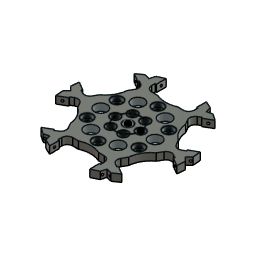
Omni_1 (Autodesk Fusion 360 design; units mm, degrees)
Autodesk Fusion 360 part; units mm, degrees
sketch "Sketch2" plane through (0, 0, 0) normal (0, 1, 0) x (1, 0, 0)
  line L0 (11.1, 32.1629) -> (11.1, 26.801)
  line L1 (-11.1, 26.801) -> (-11.1, 32.1629)
  line L2 (-11.1, 26.801) -> (-11.75, 26.801)
  line L3 (11.1, 26.801) -> (11.75, 26.801)
  line L4 (0, 0) -> (-15.82, 27.401)
  line L5 (0, 0) -> (15.82, 27.401)
  line L6 (0, 0) -> (0, 55) construction
  line L7 (15.82, 27.401) -> (15.0435, 30.2988)
  line L8 (-15.82, 27.401) -> (-15.0435, 30.2988)
  line L9 (-15.0435, 30.2988) -> (-11.1, 32.1629)
  line L10 (15.0435, 30.2988) -> (11.1, 32.1629)
  line L11 (-11.75, 26.801) -> (-11.75, 24.801)
  line L12 (11.75, 26.801) -> (11.75, 24.801)
  line L13 (-8.7379, 21.8005) -> (-5.5379, 21.8005)
  line L14 (8.7379, 21.8005) -> (5.5379, 21.8005)
  arc A0 (-11.75, 24.801) -> (-8.7379, 21.8005) centre (-8.75, 24.8004) ccw
  arc A1 (-5.5379, 21.8005) -> (5.5379, 21.8005) centre (0, 33.7826) ccw
  arc A2 (8.7379, 21.8005) -> (11.75, 24.801) centre (8.75, 24.8004) ccw
  circle A3 centre (0, 16.5) radius 1.64
  point P0 (0.1, 26.7998)
  dimension "d41" = 26.8
  dimension "d43" = 11
  dimension "d45" = 0.65
  dimension "d46" = 60
  dimension "d47" = 30
  dimension "d48" = 31.64
  dimension "d49" = 0.6
  dimension "d50" = 0.6
  dimension "d51" = 135
  dimension "d52" = 135
  dimension "d53" = 3
  dimension "d54" = 3
  dimension "d55" = 2
  dimension "d56" = 2
  dimension "d63" = 6
  dimension "d64" = 3
  dimension "d65" = 6
  dimension "d66" = 3
  dimension "d67" = 3.2
  dimension "d68" = 3.2
  dimension "d69" = 26.4
  dimension "d70" = 3.28
  dimension "d71" = 16.5
  dimension "d82" = 11.1
  dimension "d83" = 11.1
  constraint vertical L0
  constraint vertical L1
  constraint perpendicular L1 L2
  constraint perpendicular L0 L3
  constraint equal L2 L3
  constraint coincident L4.start L5.start
  constraint vertical L6
  constraint equal L4 L5
  constraint perpendicular L2 L11
  constraint perpendicular L3 L12
  constraint perpendicular L1 L13
  constraint horizontal L14
  constraint coincident L6 A3.centre
  measures "d41" distance of L4.start P0
  measures "d43" distance of L0 P0
  measures "d45" distance of L1.start L2.end
  measures "d46" angle of L4 L5
  measures "d47" angle of L5 L6
  measures "d48" distance of L4.start L4.end
  measures "d49" distance of L2 L4.end
  measures "d50" distance of L3 L5.end
  measures "d51" angle of L5 L7
  measures "d52" angle of L4 L8
  measures "d53" distance of L4.end L8.end
  measures "d54" distance of L5.end L7.end
  measures "d55" distance of L2.end L11.end
  measures "d56" distance of L3.end L12.end
  measures "d63" diameter of A0
  measures "d64" distance of L11.end A0.centre
  measures "d65" diameter of A2
  measures "d66" distance of L12.end A2.centre
  measures "d67" distance of L13.start L13.end
  measures "d68" distance of L14.start L14.end
  measures "d69" diameter of A1
  measures "d70" diameter of A3
  measures "d71" distance of L4.start A3.centre
  measures "d82" distance of L1 L6
  measures "d83" distance of L0 L6
extrude "Extrude2" add sketch "Sketch2" along normal blind 4 makes body 1
pattern_circular "C-Pattern2" count 6 over 360 about axis through (0, 1.75, 0) along (0, 1, 0) of bodies 1 makes body 2 at (-9.0005, 0, -9.4076) makes body 3 at (-12.6475, 0, 3.0909) makes body 4 at (-3.647, 0, 12.4985) makes body 5 at (9.0005, 0, 9.4076) makes body 6 at (12.6475, 0, -3.0909)
combine "Combine1" operation add target body 2 tool bodies 3 4 5 6 1
sketch "Sketch3" plane through (0, 4, 0) normal (0, 1, 0) x (-1, 0, 0)
  circle A0 centre (0, -16.5) radius 1.64
  circle A1 centre (-14.2894, -8.25) radius 1.64
  circle A2 centre (-14.2894, 8.25) radius 1.64
  circle A3 centre (0, 16.5) radius 1.64
  circle A4 centre (14.2894, 8.25) radius 1.64
  circle A5 centre (14.2894, -8.25) radius 1.64
  line L0 (28.7604, -3.7876) -> (33.4039, -6.4685)
  line L1 (33.4039, -6.4685) -> (33.7613, -2.1213)
  line L2 (33.7613, -2.1213) -> (31.64, 0)
  line L3 (31.64, 0) -> (33.7613, 2.1213)
  line L4 (33.7613, 2.1213) -> (33.4039, 6.4685)
  line L5 (33.4039, 6.4685) -> (28.7604, 3.7876)
  line L6 (28.7604, 3.7876) -> (29.0854, 3.2247)
  line L7 (29.0854, 3.2247) -> (27.3533, 2.2247)
  arc A6 (23.2487, 3.333) -> (27.3533, 2.2247) centre (25.8528, 4.8225) ccw
  line L8 (23.2487, 3.333) -> (21.6487, 6.1042)
  arc A7 (16.1108, 15.6962) -> (21.6487, 6.1042) centre (29.2566, 16.8913) ccw
  line L9 (16.1108, 15.6962) -> (14.5108, 18.4675)
  arc A8 (15.6033, 22.5763) -> (14.5108, 18.4675) centre (17.1028, 19.9779) ccw
  line L10 (15.6033, 22.5763) -> (17.3354, 23.5763)
  line L11 (17.3354, 23.5763) -> (17.6604, 23.0134)
  line L12 (17.6604, 23.0134) -> (22.3039, 25.6943)
  line L13 (22.3039, 25.6943) -> (18.7178, 28.1775)
  line L14 (18.7178, 28.1775) -> (15.82, 27.401)
  line L15 (15.82, 27.401) -> (15.0435, 30.2988)
  line L16 (15.0435, 30.2988) -> (11.1, 32.1629)
  line L17 (11.1, 32.1629) -> (11.1, 26.801)
  line L18 (11.1, 26.801) -> (11.75, 26.801)
  line L19 (11.75, 26.801) -> (11.75, 24.801)
  arc A9 (8.7379, 21.8005) -> (11.75, 24.801) centre (8.75, 24.8004) ccw
  line L20 (8.7379, 21.8005) -> (5.5379, 21.8005)
  arc A10 (-5.5379, 21.8005) -> (5.5379, 21.8005) centre (0, 33.7826) ccw
  line L21 (-5.5379, 21.8005) -> (-8.7379, 21.8005)
  arc A11 (-11.75, 24.801) -> (-8.7379, 21.8005) centre (-8.75, 24.8004) ccw
  line L22 (-11.75, 24.801) -> (-11.75, 26.801)
  line L23 (-11.75, 26.801) -> (-11.1, 26.801)
  line L24 (-11.1, 26.801) -> (-11.1, 32.1629)
  line L25 (-11.1, 32.1629) -> (-15.0435, 30.2988)
  line L26 (-15.0435, 30.2988) -> (-15.82, 27.401)
  line L27 (-15.82, 27.401) -> (-18.7178, 28.1775)
  line L28 (-18.7178, 28.1775) -> (-22.3039, 25.6943)
  line L29 (-22.3039, 25.6943) -> (-17.6604, 23.0134)
  line L30 (-17.6604, 23.0134) -> (-17.3354, 23.5763)
  line L31 (-17.3354, 23.5763) -> (-15.6033, 22.5763)
  arc A12 (-14.5108, 18.4675) -> (-15.6033, 22.5763) centre (-17.1028, 19.9779) ccw
  line L32 (-14.5108, 18.4675) -> (-16.1108, 15.6962)
  arc A13 (-21.6487, 6.1042) -> (-16.1108, 15.6962) centre (-29.2566, 16.8913) ccw
  line L33 (-21.6487, 6.1042) -> (-23.2487, 3.333)
  arc A14 (-27.3533, 2.2247) -> (-23.2487, 3.333) centre (-25.8528, 4.8225) ccw
  line L34 (-27.3533, 2.2247) -> (-29.0854, 3.2247)
  line L35 (-29.0854, 3.2247) -> (-28.7604, 3.7876)
  line L36 (-28.7604, 3.7876) -> (-33.4039, 6.4685)
  line L37 (-33.4039, 6.4685) -> (-33.7613, 2.1213)
  line L38 (-33.7613, 2.1213) -> (-31.64, 0)
  line L39 (-31.64, 0) -> (-33.7613, -2.1213)
  line L40 (-33.7613, -2.1213) -> (-33.4039, -6.4685)
  line L41 (-33.4039, -6.4685) -> (-28.7604, -3.7876)
  line L42 (-28.7604, -3.7876) -> (-29.0854, -3.2247)
  line L43 (-29.0854, -3.2247) -> (-27.3533, -2.2247)
  arc A15 (-23.2487, -3.333) -> (-27.3533, -2.2247) centre (-25.8528, -4.8225) ccw
  line L44 (-23.2487, -3.333) -> (-21.6487, -6.1042)
  arc A16 (-16.1108, -15.6962) -> (-21.6487, -6.1042) centre (-29.2566, -16.8913) ccw
  line L45 (-16.1108, -15.6962) -> (-14.5108, -18.4675)
  arc A17 (-15.6033, -22.5763) -> (-14.5108, -18.4675) centre (-17.1028, -19.9779) ccw
  line L46 (-15.6033, -22.5763) -> (-17.3354, -23.5763)
  line L47 (-17.3354, -23.5763) -> (-17.6604, -23.0134)
  line L48 (-17.6604, -23.0134) -> (-22.3039, -25.6943)
  line L49 (-22.3039, -25.6943) -> (-18.7178, -28.1775)
  line L50 (-18.7178, -28.1775) -> (-15.82, -27.401)
  line L51 (-15.82, -27.401) -> (-15.0435, -30.2988)
  line L52 (-15.0435, -30.2988) -> (-11.1, -32.1629)
  line L53 (-11.1, -32.1629) -> (-11.1, -26.801)
  line L54 (-11.1, -26.801) -> (-11.75, -26.801)
  line L55 (-11.75, -26.801) -> (-11.75, -24.801)
  arc A18 (-8.7379, -21.8005) -> (-11.75, -24.801) centre (-8.75, -24.8004) ccw
  line L56 (-8.7379, -21.8005) -> (-5.5379, -21.8005)
  arc A19 (5.5379, -21.8005) -> (-5.5379, -21.8005) centre (0, -33.7826) ccw
  line L57 (5.5379, -21.8005) -> (8.7379, -21.8005)
  arc A20 (11.75, -24.801) -> (8.7379, -21.8005) centre (8.75, -24.8004) ccw
  line L58 (11.75, -24.801) -> (11.75, -26.801)
  line L59 (11.75, -26.801) -> (11.1, -26.801)
  line L60 (11.1, -26.801) -> (11.1, -32.1629)
  line L61 (11.1, -32.1629) -> (15.0435, -30.2988)
  line L62 (15.0435, -30.2988) -> (15.82, -27.401)
  line L63 (15.82, -27.401) -> (18.7178, -28.1775)
  line L64 (18.7178, -28.1775) -> (22.3039, -25.6943)
  line L65 (22.3039, -25.6943) -> (17.6604, -23.0134)
  line L66 (17.6604, -23.0134) -> (17.3354, -23.5763)
  line L67 (17.3354, -23.5763) -> (15.6033, -22.5763)
  arc A21 (14.5108, -18.4675) -> (15.6033, -22.5763) centre (17.1028, -19.9779) ccw
  line L68 (14.5108, -18.4675) -> (16.1108, -15.6962)
  arc A22 (21.6487, -6.1042) -> (16.1108, -15.6962) centre (29.2566, -16.8913) ccw
  line L69 (21.6487, -6.1042) -> (23.2487, -3.333)
  arc A23 (27.3533, -2.2247) -> (23.2487, -3.333) centre (25.8528, -4.8225) ccw
  line L70 (27.3533, -2.2247) -> (29.0854, -3.2247)
  line L71 (29.0854, -3.2247) -> (28.7604, -3.7876)
  line L72 (0, 0) -> (15.82, 27.401) construction
  circle A24 centre (7.5, 12.9904) radius 3.5
  dimension "d76" = 15
  dimension "d77" = 7
  constraint coincident L72.start origin
  constraint coincident L14.end L15.start
  constraint coincident L72 A24.centre
  measures "d76" distance of L72.start A24.centre
  measures "d77" diameter of A24
extrude "Extrude3" cut sketch "Sketch3" against normal blind 4 contours A24 bodies 2
pattern_circular "C-Pattern3" count 6 over 360 about axis through (0, 1.75, 0) along (0, 1, 0) of "Extrude3"
ref_plane "WorkPlane1" through (0, 2, -29.482) normal (1, 0, 0) x (0, 0, -1)
sketch "Sketch4" plane through (0, 2, -29.482) normal (1, 0, 0) x (0, 0, -1)
  circle A0 centre (-0.0309, 0) radius 0.6
  line L0 (-2.6809, -2) -> (2.6809, -2) construction
  line L1 (2.6809, -2) -> (2.6809, 2) construction
  line L2 (2.6809, 2) -> (-2.6809, 2) construction
  line L3 (-2.6809, 2) -> (-2.6809, -2) construction
  dimension "d85" = 1.2
  dimension "d86" = 2.65
  measures "d85" diameter of A0
  measures "d86" distance of A0.centre L3
extrude "Extrude4" cut sketch "Sketch4" along normal blind 30 and the other way blind 30 bodies 2
pattern_circular "C-Pattern4" count 6 over 360 about axis through (0, 1.75, 0) along (0, 1, 0) of "Extrude4"
sketch "Sketch5" plane through (0, 4, 0) normal (0, 1, 0) x (-1, 0, 0)
  circle A0 centre (15, 0) radius 3.5
  circle A1 centre (7.5, -12.9904) radius 3.5
  circle A2 centre (-7.5, -12.9904) radius 3.5
  circle A3 centre (-15, 0) radius 3.5
  circle A4 centre (-7.5, 12.9904) radius 3.5
  circle A5 centre (7.5, 12.9904) radius 3.5
  circle A6 centre (0, -16.5) radius 1.64
  circle A7 centre (-14.2894, -8.25) radius 1.64
  circle A8 centre (-14.2894, 8.25) radius 1.64
  circle A9 centre (0, 16.5) radius 1.64
  circle A10 centre (14.2894, 8.25) radius 1.64
  circle A11 centre (14.2894, -8.25) radius 1.64
  line L0 (28.7604, -3.7876) -> (33.4039, -6.4685)
  line L1 (33.4039, -6.4685) -> (33.7613, -2.1213)
  line L2 (33.7613, -2.1213) -> (31.64, 0)
  line L3 (31.64, 0) -> (33.7613, 2.1213)
  line L4 (33.7613, 2.1213) -> (33.4039, 6.4685)
  line L5 (33.4039, 6.4685) -> (28.7604, 3.7876)
  line L6 (28.7604, 3.7876) -> (29.0854, 3.2247)
  line L7 (29.0854, 3.2247) -> (27.3533, 2.2247)
  arc A12 (23.2487, 3.333) -> (27.3533, 2.2247) centre (25.8528, 4.8225) ccw
  line L8 (23.2487, 3.333) -> (21.6487, 6.1042)
  arc A13 (16.1108, 15.6962) -> (21.6487, 6.1042) centre (29.2566, 16.8913) ccw
  line L9 (16.1108, 15.6962) -> (14.5108, 18.4675)
  arc A14 (15.6033, 22.5763) -> (14.5108, 18.4675) centre (17.1028, 19.9779) ccw
  line L10 (15.6033, 22.5763) -> (17.3354, 23.5763)
  line L11 (17.3354, 23.5763) -> (17.6604, 23.0134)
  line L12 (17.6604, 23.0134) -> (22.3039, 25.6943)
  line L13 (22.3039, 25.6943) -> (18.7178, 28.1775)
  line L14 (18.7178, 28.1775) -> (15.82, 27.401)
  line L15 (15.82, 27.401) -> (15.0435, 30.2988)
  line L16 (15.0435, 30.2988) -> (11.1, 32.1629)
  line L17 (11.1, 32.1629) -> (11.1, 26.801)
  line L18 (11.1, 26.801) -> (11.75, 26.801)
  line L19 (11.75, 26.801) -> (11.75, 24.801)
  arc A15 (8.7379, 21.8005) -> (11.75, 24.801) centre (8.75, 24.8004) ccw
  line L20 (8.7379, 21.8005) -> (5.5379, 21.8005)
  arc A16 (-5.5379, 21.8005) -> (5.5379, 21.8005) centre (0, 33.7826) ccw
  line L21 (-5.5379, 21.8005) -> (-8.7379, 21.8005)
  arc A17 (-11.75, 24.801) -> (-8.7379, 21.8005) centre (-8.75, 24.8004) ccw
  line L22 (-11.75, 24.801) -> (-11.75, 26.801)
  line L23 (-11.75, 26.801) -> (-11.1, 26.801)
  line L24 (-11.1, 26.801) -> (-11.1, 32.1629)
  line L25 (-11.1, 32.1629) -> (-15.0435, 30.2988)
  line L26 (-15.0435, 30.2988) -> (-15.82, 27.401)
  line L27 (-15.82, 27.401) -> (-18.7178, 28.1775)
  line L28 (-18.7178, 28.1775) -> (-22.3039, 25.6943)
  line L29 (-22.3039, 25.6943) -> (-17.6604, 23.0134)
  line L30 (-17.6604, 23.0134) -> (-17.3354, 23.5763)
  line L31 (-17.3354, 23.5763) -> (-15.6033, 22.5763)
  arc A18 (-14.5108, 18.4675) -> (-15.6033, 22.5763) centre (-17.1028, 19.9779) ccw
  line L32 (-14.5108, 18.4675) -> (-16.1108, 15.6962)
  arc A19 (-21.6487, 6.1042) -> (-16.1108, 15.6962) centre (-29.2566, 16.8913) ccw
  line L33 (-21.6487, 6.1042) -> (-23.2487, 3.333)
  arc A20 (-27.3533, 2.2247) -> (-23.2487, 3.333) centre (-25.8528, 4.8225) ccw
  line L34 (-27.3533, 2.2247) -> (-29.0854, 3.2247)
  line L35 (-29.0854, 3.2247) -> (-28.7604, 3.7876)
  line L36 (-28.7604, 3.7876) -> (-33.4039, 6.4685)
  line L37 (-33.4039, 6.4685) -> (-33.7613, 2.1213)
  line L38 (-33.7613, 2.1213) -> (-31.64, 0)
  line L39 (-31.64, 0) -> (-33.7613, -2.1213)
  line L40 (-33.7613, -2.1213) -> (-33.4039, -6.4685)
  line L41 (-33.4039, -6.4685) -> (-28.7604, -3.7876)
  line L42 (-28.7604, -3.7876) -> (-29.0854, -3.2247)
  line L43 (-29.0854, -3.2247) -> (-27.3533, -2.2247)
  arc A21 (-23.2487, -3.333) -> (-27.3533, -2.2247) centre (-25.8528, -4.8225) ccw
  line L44 (-23.2487, -3.333) -> (-21.6487, -6.1042)
  arc A22 (-16.1108, -15.6962) -> (-21.6487, -6.1042) centre (-29.2566, -16.8913) ccw
  line L45 (-16.1108, -15.6962) -> (-14.5108, -18.4675)
  arc A23 (-15.6033, -22.5763) -> (-14.5108, -18.4675) centre (-17.1028, -19.9779) ccw
  line L46 (-15.6033, -22.5763) -> (-17.3354, -23.5763)
  line L47 (-17.3354, -23.5763) -> (-17.6604, -23.0134)
  line L48 (-17.6604, -23.0134) -> (-22.3039, -25.6943)
  line L49 (-22.3039, -25.6943) -> (-18.7178, -28.1775)
  line L50 (-18.7178, -28.1775) -> (-15.82, -27.401)
  line L51 (-15.82, -27.401) -> (-15.0435, -30.2988)
  line L52 (-15.0435, -30.2988) -> (-11.1, -32.1629)
  line L53 (-11.1, -32.1629) -> (-11.1, -26.801)
  line L54 (-11.1, -26.801) -> (-11.75, -26.801)
  line L55 (-11.75, -26.801) -> (-11.75, -24.801)
  arc A24 (-8.7379, -21.8005) -> (-11.75, -24.801) centre (-8.75, -24.8004) ccw
  line L56 (-8.7379, -21.8005) -> (-5.5379, -21.8005)
  arc A25 (5.5379, -21.8005) -> (-5.5379, -21.8005) centre (0, -33.7826) ccw
  line L57 (5.5379, -21.8005) -> (8.7379, -21.8005)
  arc A26 (11.75, -24.801) -> (8.7379, -21.8005) centre (8.75, -24.8004) ccw
  line L58 (11.75, -24.801) -> (11.75, -26.801)
  line L59 (11.75, -26.801) -> (11.1, -26.801)
  line L60 (11.1, -26.801) -> (11.1, -32.1629)
  line L61 (11.1, -32.1629) -> (15.0435, -30.2988)
  line L62 (15.0435, -30.2988) -> (15.82, -27.401)
  line L63 (15.82, -27.401) -> (18.7178, -28.1775)
  line L64 (18.7178, -28.1775) -> (22.3039, -25.6943)
  line L65 (22.3039, -25.6943) -> (17.6604, -23.0134)
  line L66 (17.6604, -23.0134) -> (17.3354, -23.5763)
  line L67 (17.3354, -23.5763) -> (15.6033, -22.5763)
  arc A27 (14.5108, -18.4675) -> (15.6033, -22.5763) centre (17.1028, -19.9779) ccw
  line L68 (14.5108, -18.4675) -> (16.1108, -15.6962)
  arc A28 (21.6487, -6.1042) -> (16.1108, -15.6962) centre (29.2566, -16.8913) ccw
  line L69 (21.6487, -6.1042) -> (23.2487, -3.333)
  arc A29 (27.3533, -2.2247) -> (23.2487, -3.333) centre (25.8528, -4.8225) ccw
  line L70 (27.3533, -2.2247) -> (29.0854, -3.2247)
  line L71 (29.0854, -3.2247) -> (28.7604, -3.7876)
  circle A30 centre (0, 0) radius 2.6
  circle A31 centre (-7, 0) radius 2.5
  circle A32 centre (0, 0) radius 7 construction
  circle A33 centre (0, 0) radius 7 construction
  circle A34 centre (-3.5, -6.0622) radius 2.5
  circle A35 centre (0, 0) radius 7 construction
  circle A36 centre (3.5, -6.0622) radius 2.5
  circle A37 centre (0, 0) radius 7 construction
  circle A38 centre (7, 0) radius 2.5
  circle A39 centre (0, 0) radius 7 construction
  circle A40 centre (3.5, 6.0622) radius 2.5
  circle A41 centre (0, 0) radius 7 construction
  circle A42 centre (-3.5, 6.0622) radius 2.5
  circle A43 centre (0, -16.5) radius 3
  circle A44 centre (14.2894, -8.25) radius 3
  circle A45 centre (14.2894, 8.25) radius 3
  circle A46 centre (0, 16.5) radius 3
  circle A47 centre (-14.2894, 8.25) radius 3
  circle A48 centre (-14.2894, -8.25) radius 3
  dimension "d93" = 5.2
  dimension "d96" = 5
  dimension "d98" = 360
  dimension "d101" = 6
  dimension "d103" = 360
  dimension "d104" = 14
  constraint coincident A30.centre A32.centre
  constraint concentric A30 A32
  constraint coincident A31.centre A32
  constraint concentric A6 A43
  constraint horizontal A31.centre A38.centre
  measures "d93" diameter of A30
  measures "d96" diameter of A31
  measures "d101" diameter of A43
  measures "d104" diameter of A41
extrude "Extrude5" cut sketch "Sketch5" against normal blind 4 contours A30 bodies 2
extrude "Extrude6" cut sketch "Sketch5" against normal blind 4 contours A31 | A34 | A36 | A38 | A40 | A42 bodies 2
extrude "Extrude7" cut sketch "Sketch5" against normal blind 2.5 contours A43 | A44 | A45 | A46 | A47 | A48 bodies 2
equation "d50 = d49"
equation "d54 = d53"
equation "d83 = d82"
equation "d84 = d82"
